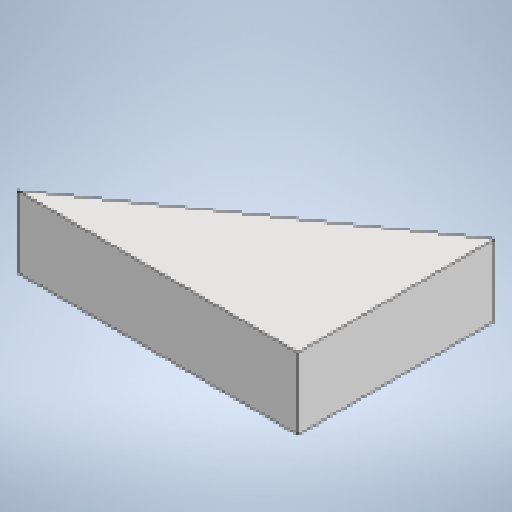
# Autodesk Inventor part: NDM-VOS dummy upstairse
Saved by Autodesk Inventor 2025 (Build 290162010, 162A)
## iProperties
Created: 2024-10-13
Part Number: NDM-VOS dummy upstairse
Material: Generic
Document SubType Name: Modeling
Designer: admin
Density: 1 g/cm^3
Appearance: Default
Author: admin
Autodesk Inventor part; units mm, degrees
ref_plane "YZ Plane" through (0, 0, 0) normal (1, 0, 0) x (0, 1, 0)
ref_plane "XZ Plane" through (0, 0, 0) normal (0, 1, 0) x (-1, 0, 0)
ref_plane "XY Plane" through (0, 0, 0) normal (0, 0, 1) x (1, 0, 0)
sketch "Sketch1" plane through (0, 0, 0) normal (0, 0, 1) x (1, 0, 0)
  line L0 (0, 0) -> (0, 2200)
  line L1 (0, 2200) -> (-3141.9256, 0)
  line L2 (-3141.9256, 0) -> (0, 0)
  dimension "d0" = 2200
  dimension "d1" = 35
  constraints: 6 end point, 1 perpendicular, 1 vertical
  measures "d0" distance of L0.start L0.end
  measures "d1" angle of L2 L1
extrude "Extrusion1" add sketch "Sketch1" along normal mid plane 800
body "Solid1"
